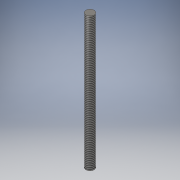
# Autodesk Inventor part: Piston Lead screw M8
Saved by Autodesk Inventor 2018 (Build 220112000, 112)
## iProperties
Created: 2013-10-18
Part Number: Piston Lead screw M8
Material: Steel, Carbon
Document SubType Name: Modeling
Designer: Gabriel Smolnycki
Mass: 51.2959 g
Surface Area: 33.6779 cm^2
Volume: 6.53451 cm^3
Density: 7.85 g/cm^3
Appearance: Semi-Polished
Sending System: SolidWorks 2017
Last Author: Gabriel Smolnycki
Last Saved: 2017-09-14
Author: Gabriel Smolnycki
Autodesk Inventor part; units mm, degrees
ref_plane "YZ Plane" through (0, 0, 0) normal (1, 0, 0) x (0, 1, 0)
ref_plane "XY Plane" through (0, 0, 0) normal (0, 0, 1) x (1, 0, 0)
ref_plane "Work Plane1" through (0, -130, 0) normal (0, 1, 0) x (-1, 0, 0)
sketch "Sketch1" plane through (0, -130, 0) normal (0, 1, 0) x (-1, 0, 0)
  circle A0 centre (0, 0) radius 4
  constraints: 1 centre point
extrude "Extrusion1" add sketch "Sketch1" along normal blind 130
thread "Thread1" size "TR8x1.5" class "7e" standard "ISO Metric Trapezoidal Threads" full length
body "Solid3"
